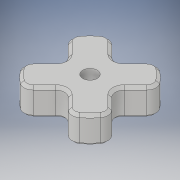
# Autodesk Inventor part: Top Part
Saved by Autodesk Inventor 2019 (Build 230136000, 136)
## iProperties
Created: 2019-01-02
Part Number: Top Part
Material: Generic
Document SubType Name: Modeling
Designer: spike
Density: 1 g/cm^3
Appearance: Default
Author: spike
Autodesk Inventor part; units mm, degrees
note: some values were not read from the file. Chosen so that the rebuilt part matches the saved one: sketch regions of "Extrusion8".
ref_plane "YZ Plane" through (0, 0, 0) normal (1, 0, 0) x (0, 1, 0)
ref_plane "XZ Plane" through (0, 0, 0) normal (0, 1, 0) x (-1, 0, 0)
ref_plane "XY Plane" through (0, 0, 0) normal (0, 0, 1) x (1, 0, 0)
sketch "Sketch1" plane through (0, 0, 0) normal (0, 1, 0) x (-1, 0, 0)
  circle A0 centre (0, 0) radius 11
  circle A1 centre (0, 0) radius 4
  line L0 (8.0829, 0) -> (4.0415, -7)
  line L1 (4.0415, -7) -> (-4.0415, -7)
  line L2 (-4.0415, -7) -> (-8.0829, 0)
  line L3 (-8.0829, 0) -> (-4.0415, 7)
  line L4 (-4.0415, 7) -> (4.0415, 7)
  line L5 (4.0415, 7) -> (8.0829, 0)
  circle A2 centre (0, 0) radius 27.5
  circle A3 centre (0, 0) radius 32.5
  line L6 (-24.5036, -24.5036) -> (24.5036, -24.5036) construction
  line L7 (24.5036, -24.5036) -> (24.5036, 24.5036) construction
  line L8 (24.5036, 24.5036) -> (-24.5036, 24.5036) construction
  line L9 (-24.5036, 24.5036) -> (-24.5036, -24.5036) construction
  line L10 (-24.5036, -24.5036) -> (24.5036, 24.5036) construction
  line L11 (24.5036, -24.5036) -> (-24.5036, 24.5036) construction
  line L12 (24.5036, 12.4828) -> (-12.4828, -24.5036)
  line L13 (12.4828, 24.5036) -> (-24.5036, -12.4828)
  line L14 (-12.4828, 24.5036) -> (24.5036, -12.4828)
  line L15 (12.4828, -24.5036) -> (-24.5036, 12.4828)
  circle A4 centre (0, 0) radius 9
  dimension "d3" = 55
  dimension "d0" = 22
  dimension "d1" = 8
  dimension "d2" = 14
  dimension "d4" = 65
  dimension "d5" = 17
  dimension "d12" = 2
  constraints: 32 end point, 8 point on line, 6 coincident, 4 centre point, 2 midpoint, 2 parallel, 2 perpendicular, 1 horizontal, 23 other
  measures "d0" diameter of A0
  measures "d1" diameter of A1
  measures "d2" distance between parallel lines of L3 L0
  measures "d4" diameter of A3
  measures "d5" distance between parallel lines of L15 L14
  measures "d12" radial gap between concentric circles of A0 A4
extrude "Extrusion8" add sketch "Sketch1" along normal blind 15 contours A0 L12 A4 L14 | A0 L14 L12 | L14 A4 A0 | A0 L14 L13 A2 L12 | L12 L14 A2 L15 A0 | A0 L12 A4 | L14 A4 L13 A0 | A0 L13 L14 | A4 L12 L15 L13 L14 | L14 A4 | L12 L15 A0 | A0 L15 A4 L12 | A4 L12 | L13 A4 A0 | A0 L13 L15 A2 L14 | L15 L12 A2 L13 A0 | A0 L15 A4 | L13 A4 L15 A0 | A0 L15 L13 | L13 A4 | A4 L15 | L0 L1 L2 L3 L4 L5
fillet "Fillet3" radius 5 12 edges at (24.5036, 7.5, -12.4828) (12.0208, 7.5, 0) (24.5036, 7.5, 12.4828) (12.4828, 7.5, 24.5036) (0, 7.5, 12.0208) (-12.4828, 7.5, 24.5036) (-24.5036, 7.5, 12.4828) (-12.0208, 7.5, 0) (-24.5036, 7.5, -12.4828) (-12.4828, 7.5, -24.5036) (0, 7.5, -12.0208) (12.4828, 7.5, -24.5036)
chamfer "Chamfer3" distance 1.5 angle 45 48 edges at (18.6415, 15, 6.6207) (14.0919, 15, 0) (18.6415, 15, -6.6207) (23.1759, 15, -12.8513) (19.4454, 15, -19.4454) (12.8513, 15, -23.1759) (6.6207, 15, -18.6415) (0, 15, -14.0919) (-6.6207, 15, -18.6415) (-12.8513, 15, -23.1759) (-19.4454, 15, -19.4454) (-23.1759, 15, -12.8513) (-18.6415, 15, -6.6207) (-14.0919, 15, 0) (-18.6415, 15, 6.6207) (-23.1759, 15, 12.8513) (-19.4454, 15, 19.4454) (-12.8513, 15, 23.1759) (-6.6207, 15, 18.6415) (0, 15, 14.0919) (6.6207, 15, 18.6415) (12.8513, 15, 23.1759) (19.4454, 15, 19.4454) (23.1759, 15, 12.8513) (0, 0, -14.0919) (-6.6207, 0, -18.6415) (-12.8513, 0, -23.1759) (-19.4454, 0, -19.4454) (-23.1759, 0, -12.8513) (-18.6415, 0, -6.6207) (-14.0919, 0, 0) (-18.6415, 0, 6.6207) (-23.1759, 0, 12.8513) (-19.4454, 0, 19.4454) (-12.8513, 0, 23.1759) (-6.6207, 0, 18.6415) (0, 0, 14.0919) (6.6207, 0, 18.6415) (12.8513, 0, 23.1759) (19.4454, 0, 19.4454) (23.1759, 0, 12.8513) (18.6415, 0, 6.6207) (14.0919, 0, 0) (18.6415, 0, -6.6207) (23.1759, 0, -12.8513) (19.4454, 0, -19.4454) (12.8513, 0, -23.1759) (6.6207, 0, -18.6415)
extrude "Extrusion9" cut sketch "Sketch1" along normal blind 6 contours L0 L1 L2 L3 L4 L5
equation "\"d3\" = SpacerDiameter"
equation "\"d0\" = BearingDiameter"
equation "\"d1\" = RodDiameter"
equation "\"d2\" = NutDiameter"
equation "\"d4\" = SpacerDiameter + LipDepth"
equation "\"d29\" = SpacerHeight"
equation "\"d35\" = NutHeight"
equation "\"RodDiameter\" = 8"
equation "\"NutDiameter\" = 14"
equation "\"NutHeight\" = 6"
equation "\"SpacerHeight\" = 15"
equation "\"SpacerDiameter\" = 55"
equation "\"LipDepth\" = 10"
equation "\"BearingHeight\" = 7"
equation "\"BearingDiameter\" = 22"
body "Solid3"
